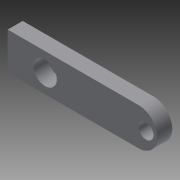
# Autodesk Inventor part: handle_crank
Saved by Autodesk Inventor 2016 (Build 200138000, 138)
## iProperties
Created: 2015-09-10
Part Number: handle_crank
Material: Generic
Document SubType Name: Modeling
Designer: Students
Density: 1 g/cm^3
Appearance: Default
Author: Students
Autodesk Inventor part; units mm, degrees
ref_plane "YZ Plane" through (0, 0, 0) normal (1, 0, 0) x (0, 1, 0)
ref_plane "XZ Plane" through (0, 0, 0) normal (0, 1, 0) x (-1, 0, 0)
ref_plane "XY Plane" through (0, 0, 0) normal (0, 0, 1) x (1, 0, 0)
sketch "Sketch1" plane through (0, 0, 0) normal (0, 1, 0) x (-1, 0, 0)
  line L0 (0, 0) -> (87.5, 0)
  line L1 (87.5, 0) -> (87.5, 25)
  line L2 (87.5, 25) -> (0, 25)
  circle A0 centre (62.5, 12.5) radius 7.8
  arc A1 (0, 25) -> (0, 0) centre (0, 12.5) ccw
  circle A2 centre (-5, 12.5) radius 5
  constraints: 6 coincident, 6 end point, 3 centre point, 2 point on circle, 1 horizontal, 1 parallel, 1 perpendicular
extrude "Extrusion1" add sketch "Sketch1" along normal blind 10
body "Solid1"
